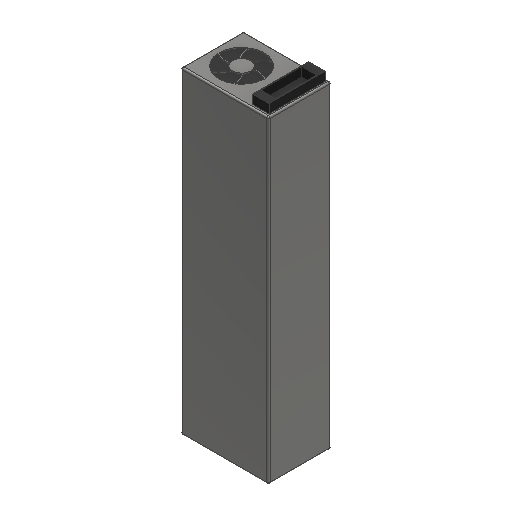
# Autodesk Inventor part: COTS_HP_DPS-600PB_PSU
Saved by Autodesk Inventor 2026.1 (Build 301233000, 233)
## iProperties
Created: 2016-06-20
Part Number: COTS_HP_DPS-600PB_PSU
Material: Ogólny
Document SubType Name: Modeling
Designer: Andrzej
Density: 1 g/cm^3
Appearance: Anodowana - jasnoszara
Author: Andrzej
Autodesk Inventor part; units mm, degrees
(part 1 of 2)
ref_plane "YZ Plane" through (0, 0, 0) normal (1, 0, 0) x (0, 1, 0)
ref_plane "XZ Plane" through (0, 0, 0) normal (0, 1, 0) x (-1, 0, 0)
ref_plane "XY Plane" through (0, 0, 0) normal (0, 0, 1) x (1, 0, 0)
sketch "Szkic1" plane through (0, 0, 0) normal (0, 0, 1) x (1, 0, 0)
  line L0 (-0.3998, -24.5096) -> (77.1002, -24.5096)
  line L1 (77.1002, -24.5096) -> (77.1002, -80.0096)
  line L2 (77.1002, -80.0096) -> (-0.3998, -80.0096)
  line L3 (-0.3998, -80.0096) -> (-0.3998, -24.5096)
  point P0 (0, 0)
  dimension "d0" = 77.5
  dimension "d1" = 55.5
  constraints: 8 end point, 2 parallel, 1 horizontal, 1 perpendicular
  measures "d0" distance of L1.end L2.end
  measures "d1" distance of L0.end L1.end
extrude "Wyciągnięcie proste1" add sketch "Szkic1" along normal blind 281.5
fillet "Zaokrąglenie1" radius 1.5 12 edges at (77.1002, -24.5096, 140.75) (77.1002, -80.0096, 140.75) (-0.3998, -24.5096, 140.75) (38.3502, -24.5096, 0) (38.3502, -80.0096, 0) (77.1002, -52.2596, 0) (-0.3998, -52.2596, 0) (38.3502, -24.5096, 281.5) (77.1002, -52.2596, 281.5) (38.3502, -80.0096, 281.5) (-0.3998, -52.2596, 281.5) (-0.3998, -80.0096, 140.75)
sketch "Szkic2" plane through (0, 0, 0) normal (0, 0, -1) x (-1, 0, 0)
  line L0 (-34.6002, -49.0096) -> (-3.6002, -49.0096)
  line L1 (-3.6002, -49.0096) -> (-3.6002, -73.0096)
  line L2 (-3.6002, -73.0096) -> (-34.6002, -73.0096)
  line L3 (-34.6002, -73.0096) -> (-34.6002, -49.0096)
  arc A0 (-75.6002, -24.5096) -> (-77.1002, -26.0096) centre (-75.6002, -26.0096) ccw projected
  line L4 (-77.1002, -78.5096) -> (-75.6002, -78.5096) projected
  line L5 (-75.6002, -78.5096) -> (-75.6002, -26.0096) projected
  line L6 (-75.6002, -26.0096) -> (-77.1002, -26.0096) projected
  line L7 (-77.1002, -26.0096) -> (-77.1002, -78.5096) projected
  line L8 (-75.6002, -24.5096) -> (-75.6002, -26.0096) projected
  line L9 (-75.6002, -26.0096) -> (-1.1002, -26.0096) projected
  line L10 (-1.1002, -26.0096) -> (-1.1002, -24.5096) projected
  line L11 (-1.1002, -24.5096) -> (-75.6002, -24.5096) projected
  line L12 (-1.1002, -80.0096) -> (-1.1002, -78.5096) projected
  line L13 (-1.1002, -78.5096) -> (-75.6002, -78.5096) projected
  line L14 (-75.6002, -78.5096) -> (-75.6002, -80.0096) projected
  line L15 (-75.6002, -80.0096) -> (-1.1002, -80.0096) projected
  arc A1 (-1.1002, -80.0096) -> (0.3998, -78.5096) centre (-1.1002, -78.5096) ccw projected
  line L16 (0.3998, -78.5096) -> (-1.1002, -78.5096) projected
  line L17 (0.3998, -78.5096) -> (0.3998, -26.0096) projected
  line L18 (-1.1002, -26.0096) -> (-1.1002, -78.5096) projected
  line L19 (0.3998, -26.0096) -> (-1.1002, -26.0096) projected
  line L20 (-1.1002, -26.0096) -> (-1.1002, -78.5096) projected
  line L21 (-1.1002, -78.5096) -> (0.3998, -78.5096) projected
  line L22 (0.3998, -78.5096) -> (0.3998, -26.0096) projected
  arc A2 (0.3998, -26.0096) -> (-1.1002, -24.5096) centre (-1.1002, -26.0096) ccw projected
  line L23 (-75.6002, -80.0096) -> (-75.6002, -78.5096) projected
  line L24 (-75.6002, -78.5096) -> (-75.6002, -80.0096) projected
  line L25 (-77.1002, -78.5096) -> (-75.6002, -78.5096) projected
  arc A3 (-77.1002, -78.5096) -> (-75.6002, -80.0096) centre (-75.6002, -78.5096) ccw projected
  circle A4 centre (-38.6002, -71.0096) radius 3.75
  circle A5 centre (-38.6002, -71.0096) radius 2.5
  line L26 (-31.6002, -53.0096) -> (-6.6002, -53.0096)
  line L27 (-31.6002, -69.0096) -> (-6.6002, -69.0096)
  line L28 (-31.6002, -53.0096) -> (-31.6002, -69.0096)
  line L29 (-6.6002, -53.0096) -> (-6.6002, -69.0096)
  line L30 (-70.6002, -30.3756) -> (-72.1002, -31.2416)
  line L31 (-72.1002, -31.2416) -> (-73.6002, -30.3756)
  line L32 (-73.6002, -30.3756) -> (-73.6002, -28.6435)
  line L33 (-73.6002, -28.6435) -> (-72.1002, -27.7775)
  line L34 (-72.1002, -27.7775) -> (-70.6002, -28.6435)
  line L35 (-70.6002, -28.6435) -> (-70.6002, -30.3756)
  line L36 (-68.1002, -31.2416) -> (-69.6002, -30.3756)
  line L37 (-66.6002, -30.3756) -> (-68.1002, -31.2416)
  line L38 (-69.6002, -30.3756) -> (-69.6002, -28.6435)
  line L39 (-66.6002, -28.6435) -> (-66.6002, -30.3756)
  line L40 (-69.6002, -28.6435) -> (-68.1002, -27.7775)
  line L41 (-68.1002, -27.7775) -> (-66.6002, -28.6435)
  line L42 (-64.1002, -31.2416) -> (-65.6002, -30.3756)
  line L43 (-62.6002, -30.3756) -> (-64.1002, -31.2416)
  line L44 (-65.6002, -30.3756) -> (-65.6002, -28.6435)
  line L45 (-62.6002, -28.6435) -> (-62.6002, -30.3756)
  line L46 (-65.6002, -28.6435) -> (-64.1002, -27.7775)
  line L47 (-64.1002, -27.7775) -> (-62.6002, -28.6435)
  line L48 (-60.1002, -31.2416) -> (-61.6002, -30.3756)
  line L49 (-58.6002, -30.3756) -> (-60.1002, -31.2416)
  line L50 (-61.6002, -30.3756) -> (-61.6002, -28.6435)
  line L51 (-58.6002, -28.6435) -> (-58.6002, -30.3756)
  line L52 (-61.6002, -28.6435) -> (-60.1002, -27.7775)
  line L53 (-60.1002, -27.7775) -> (-58.6002, -28.6435)
  line L54 (-56.1002, -31.2416) -> (-57.6002, -30.3756)
  line L55 (-54.6002, -30.3756) -> (-56.1002, -31.2416)
  line L56 (-57.6002, -30.3756) -> (-57.6002, -28.6435)
  line L57 (-54.6002, -28.6435) -> (-54.6002, -30.3756)
  line L58 (-57.6002, -28.6435) -> (-56.1002, -27.7775)
  line L59 (-56.1002, -27.7775) -> (-54.6002, -28.6435)
  line L60 (-52.1002, -31.2416) -> (-53.6002, -30.3756)
  line L61 (-50.6002, -30.3756) -> (-52.1002, -31.2416)
  line L62 (-53.6002, -30.3756) -> (-53.6002, -28.6435)
  line L63 (-50.6002, -28.6435) -> (-50.6002, -30.3756)
  line L64 (-53.6002, -28.6435) -> (-52.1002, -27.7775)
  line L65 (-52.1002, -27.7775) -> (-50.6002, -28.6435)
  line L66 (-48.1002, -31.2416) -> (-49.6002, -30.3756)
  line L67 (-46.6002, -30.3756) -> (-48.1002, -31.2416)
  line L68 (-49.6002, -30.3756) -> (-49.6002, -28.6435)
  line L69 (-46.6002, -28.6435) -> (-46.6002, -30.3756)
  line L70 (-49.6002, -28.6435) -> (-48.1002, -27.7775)
  line L71 (-48.1002, -27.7775) -> (-46.6002, -28.6435)
  line L72 (-44.1002, -31.2416) -> (-45.6002, -30.3756)
  line L73 (-42.6002, -30.3756) -> (-44.1002, -31.2416)
  line L74 (-45.6002, -30.3756) -> (-45.6002, -28.6435)
  line L75 (-42.6002, -28.6435) -> (-42.6002, -30.3756)
  line L76 (-45.6002, -28.6435) -> (-44.1002, -27.7775)
  line L77 (-44.1002, -27.7775) -> (-42.6002, -28.6435)
  line L78 (-40.1002, -31.2416) -> (-41.6002, -30.3756)
  line L79 (-38.6002, -30.3756) -> (-40.1002, -31.2416)
  line L80 (-41.6002, -30.3756) -> (-41.6002, -28.6435)
  line L81 (-38.6002, -28.6435) -> (-38.6002, -30.3756)
  line L82 (-41.6002, -28.6435) -> (-40.1002, -27.7775)
  line L83 (-40.1002, -27.7775) -> (-38.6002, -28.6435)
  line L84 (-36.1002, -31.2416) -> (-37.6002, -30.3756)
  line L85 (-34.6002, -30.3756) -> (-36.1002, -31.2416)
  line L86 (-37.6002, -30.3756) -> (-37.6002, -28.6435)
  line L87 (-34.6002, -28.6435) -> (-34.6002, -30.3756)
  line L88 (-37.6002, -28.6435) -> (-36.1002, -27.7775)
  line L89 (-36.1002, -27.7775) -> (-34.6002, -28.6435)
  line L90 (-32.1002, -31.2416) -> (-33.6002, -30.3756)
  line L91 (-30.6002, -30.3756) -> (-32.1002, -31.2416)
  line L92 (-33.6002, -30.3756) -> (-33.6002, -28.6435)
  line L93 (-30.6002, -28.6435) -> (-30.6002, -30.3756)
  line L94 (-33.6002, -28.6435) -> (-32.1002, -27.7775)
  line L95 (-32.1002, -27.7775) -> (-30.6002, -28.6435)
  line L96 (-28.1002, -31.2416) -> (-29.6002, -30.3756)
  line L97 (-26.6002, -30.3756) -> (-28.1002, -31.2416)
  line L98 (-29.6002, -30.3756) -> (-29.6002, -28.6435)
  line L99 (-26.6002, -28.6435) -> (-26.6002, -30.3756)
  line L100 (-29.6002, -28.6435) -> (-28.1002, -27.7775)
  line L101 (-28.1002, -27.7775) -> (-26.6002, -28.6435)
  line L102 (-24.1002, -31.2416) -> (-25.6002, -30.3756)
  line L103 (-22.6002, -30.3756) -> (-24.1002, -31.2416)
  line L104 (-25.6002, -30.3756) -> (-25.6002, -28.6435)
  line L105 (-22.6002, -28.6435) -> (-22.6002, -30.3756)
  line L106 (-25.6002, -28.6435) -> (-24.1002, -27.7775)
  line L107 (-24.1002, -27.7775) -> (-22.6002, -28.6435)
  line L108 (-20.1002, -31.2416) -> (-21.6002, -30.3756)
  line L109 (-18.6002, -30.3756) -> (-20.1002, -31.2416)
  line L110 (-21.6002, -30.3756) -> (-21.6002, -28.6435)
  line L111 (-18.6002, -28.6435) -> (-18.6002, -30.3756)
  line L112 (-21.6002, -28.6435) -> (-20.1002, -27.7775)
  line L113 (-20.1002, -27.7775) -> (-18.6002, -28.6435)
  line L114 (-16.1002, -31.2416) -> (-17.6002, -30.3756)
  line L115 (-14.6002, -30.3756) -> (-16.1002, -31.2416)
  line L116 (-17.6002, -30.3756) -> (-17.6002, -28.6435)
  line L117 (-14.6002, -28.6435) -> (-14.6002, -30.3756)
  line L118 (-17.6002, -28.6435) -> (-16.1002, -27.7775)
  line L119 (-16.1002, -27.7775) -> (-14.6002, -28.6435)
  line L120 (-12.1002, -31.2416) -> (-13.6002, -30.3756)
  line L121 (-10.6002, -30.3756) -> (-12.1002, -31.2416)
  line L122 (-13.6002, -30.3756) -> (-13.6002, -28.6435)
  line L123 (-10.6002, -28.6435) -> (-10.6002, -30.3756)
  line L124 (-13.6002, -28.6435) -> (-12.1002, -27.7775)
  line L125 (-12.1002, -27.7775) -> (-10.6002, -28.6435)
  line L126 (-8.1002, -31.2416) -> (-9.6002, -30.3756)
  line L127 (-6.6002, -30.3756) -> (-8.1002, -31.2416)
  line L128 (-9.6002, -30.3756) -> (-9.6002, -28.6435)
  line L129 (-6.6002, -28.6435) -> (-6.6002, -30.3756)
  line L130 (-9.6002, -28.6435) -> (-8.1002, -27.7775)
  line L131 (-8.1002, -27.7775) -> (-6.6002, -28.6435)
  line L132 (-72.1002, -35.2416) -> (-73.6002, -34.3756)
  line L133 (-70.6002, -34.3756) -> (-72.1002, -35.2416)
  line L134 (-73.6002, -34.3756) -> (-73.6002, -32.6435)
  line L135 (-70.6002, -32.6435) -> (-70.6002, -34.3756)
  line L136 (-73.6002, -32.6435) -> (-72.1002, -31.7775)
  line L137 (-72.1002, -31.7775) -> (-70.6002, -32.6435)
  line L138 (-68.1002, -35.2416) -> (-69.6002, -34.3756)
  line L139 (-66.6002, -34.3756) -> (-68.1002, -35.2416)
  line L140 (-69.6002, -34.3756) -> (-69.6002, -32.6435)
  line L141 (-66.6002, -32.6435) -> (-66.6002, -34.3756)
  line L142 (-69.6002, -32.6435) -> (-68.1002, -31.7775)
  line L143 (-68.1002, -31.7775) -> (-66.6002, -32.6435)
  line L144 (-64.1002, -35.2416) -> (-65.6002, -34.3756)
  line L145 (-62.6002, -34.3756) -> (-64.1002, -35.2416)
  line L146 (-65.6002, -34.3756) -> (-65.6002, -32.6435)
  line L147 (-62.6002, -32.6435) -> (-62.6002, -34.3756)
  line L148 (-65.6002, -32.6435) -> (-64.1002, -31.7775)
  line L149 (-64.1002, -31.7775) -> (-62.6002, -32.6435)
  line L150 (-60.1002, -35.2416) -> (-61.6002, -34.3756)
  line L151 (-58.6002, -34.3756) -> (-60.1002, -35.2416)
  line L152 (-61.6002, -34.3756) -> (-61.6002, -32.6435)
  line L153 (-58.6002, -32.6435) -> (-58.6002, -34.3756)
  line L154 (-61.6002, -32.6435) -> (-60.1002, -31.7775)
  line L155 (-60.1002, -31.7775) -> (-58.6002, -32.6435)
  line L156 (-56.1002, -35.2416) -> (-57.6002, -34.3756)
  line L157 (-54.6002, -34.3756) -> (-56.1002, -35.2416)
  line L158 (-57.6002, -34.3756) -> (-57.6002, -32.6435)
  line L159 (-54.6002, -32.6435) -> (-54.6002, -34.3756)
  line L160 (-57.6002, -32.6435) -> (-56.1002, -31.7775)
  line L161 (-56.1002, -31.7775) -> (-54.6002, -32.6435)
  line L162 (-52.1002, -35.2416) -> (-53.6002, -34.3756)
  line L163 (-50.6002, -34.3756) -> (-52.1002, -35.2416)
  line L164 (-53.6002, -34.3756) -> (-53.6002, -32.6435)
  line L165 (-50.6002, -32.6435) -> (-50.6002, -34.3756)
  line L166 (-53.6002, -32.6435) -> (-52.1002, -31.7775)
  line L167 (-52.1002, -31.7775) -> (-50.6002, -32.6435)
  line L168 (-48.1002, -35.2416) -> (-49.6002, -34.3756)
  line L169 (-46.6002, -34.3756) -> (-48.1002, -35.2416)
  line L170 (-49.6002, -34.3756) -> (-49.6002, -32.6435)
  line L171 (-46.6002, -32.6435) -> (-46.6002, -34.3756)
  line L172 (-49.6002, -32.6435) -> (-48.1002, -31.7775)
  line L173 (-48.1002, -31.7775) -> (-46.6002, -32.6435)
  line L174 (-44.1002, -35.2416) -> (-45.6002, -34.3756)
  line L175 (-42.6002, -34.3756) -> (-44.1002, -35.2416)
  line L176 (-45.6002, -34.3756) -> (-45.6002, -32.6435)
  line L177 (-42.6002, -32.6435) -> (-42.6002, -34.3756)
  line L178 (-45.6002, -32.6435) -> (-44.1002, -31.7775)
  line L179 (-44.1002, -31.7775) -> (-42.6002, -32.6435)
  line L180 (-40.1002, -35.2416) -> (-41.6002, -34.3756)
  line L181 (-38.6002, -34.3756) -> (-40.1002, -35.2416)
  line L182 (-41.6002, -34.3756) -> (-41.6002, -32.6435)
  line L183 (-38.6002, -32.6435) -> (-38.6002, -34.3756)
  line L184 (-41.6002, -32.6435) -> (-40.1002, -31.7775)
  line L185 (-40.1002, -31.7775) -> (-38.6002, -32.6435)
  line L186 (-36.1002, -35.2416) -> (-37.6002, -34.3756)
  line L187 (-34.6002, -34.3756) -> (-36.1002, -35.2416)
  line L188 (-37.6002, -34.3756) -> (-37.6002, -32.6435)
  line L189 (-34.6002, -32.6435) -> (-34.6002, -34.3756)
  line L190 (-37.6002, -32.6435) -> (-36.1002, -31.7775)
  line L191 (-36.1002, -31.7775) -> (-34.6002, -32.6435)
  line L192 (-32.1002, -35.2416) -> (-33.6002, -34.3756)
  line L193 (-30.6002, -34.3756) -> (-32.1002, -35.2416)
  line L194 (-33.6002, -34.3756) -> (-33.6002, -32.6435)
  line L195 (-30.6002, -32.6435) -> (-30.6002, -34.3756)
  line L196 (-33.6002, -32.6435) -> (-32.1002, -31.7775)
  line L197 (-32.1002, -31.7775) -> (-30.6002, -32.6435)
  line L198 (-28.1002, -35.2416) -> (-29.6002, -34.3756)
  line L199 (-26.6002, -34.3756) -> (-28.1002, -35.2416)
  line L200 (-29.6002, -34.3756) -> (-29.6002, -32.6435)
  line L201 (-26.6002, -32.6435) -> (-26.6002, -34.3756)
  line L202 (-29.6002, -32.6435) -> (-28.1002, -31.7775)
  line L203 (-28.1002, -31.7775) -> (-26.6002, -32.6435)
  line L204 (-24.1002, -35.2416) -> (-25.6002, -34.3756)
  line L205 (-22.6002, -34.3756) -> (-24.1002, -35.2416)
  line L206 (-25.6002, -34.3756) -> (-25.6002, -32.6435)
  line L207 (-22.6002, -32.6435) -> (-22.6002, -34.3756)
  line L208 (-25.6002, -32.6435) -> (-24.1002, -31.7775)
  line L209 (-24.1002, -31.7775) -> (-22.6002, -32.6435)
  line L210 (-20.1002, -35.2416) -> (-21.6002, -34.3756)
  line L211 (-18.6002, -34.3756) -> (-20.1002, -35.2416)
  line L212 (-21.6002, -34.3756) -> (-21.6002, -32.6435)
  line L213 (-18.6002, -32.6435) -> (-18.6002, -34.3756)
  line L214 (-21.6002, -32.6435) -> (-20.1002, -31.7775)
  line L215 (-20.1002, -31.7775) -> (-18.6002, -32.6435)
  line L216 (-16.1002, -35.2416) -> (-17.6002, -34.3756)
  line L217 (-14.6002, -34.3756) -> (-16.1002, -35.2416)
  line L218 (-17.6002, -34.3756) -> (-17.6002, -32.6435)
  line L219 (-14.6002, -32.6435) -> (-14.6002, -34.3756)
  line L220 (-17.6002, -32.6435) -> (-16.1002, -31.7775)
  line L221 (-16.1002, -31.7775) -> (-14.6002, -32.6435)
  line L222 (-12.1002, -35.2416) -> (-13.6002, -34.3756)
  line L223 (-10.6002, -34.3756) -> (-12.1002, -35.2416)
  line L224 (-13.6002, -34.3756) -> (-13.6002, -32.6435)
  line L225 (-10.6002, -32.6435) -> (-10.6002, -34.3756)
  line L226 (-13.6002, -32.6435) -> (-12.1002, -31.7775)
  line L227 (-12.1002, -31.7775) -> (-10.6002, -32.6435)
  line L228 (-8.1002, -35.2416) -> (-9.6002, -34.3756)
  line L229 (-6.6002, -34.3756) -> (-8.1002, -35.2416)
  line L230 (-9.6002, -34.3756) -> (-9.6002, -32.6435)
  line L231 (-6.6002, -32.6435) -> (-6.6002, -34.3756)
  line L232 (-9.6002, -32.6435) -> (-8.1002, -31.7775)
  line L233 (-8.1002, -31.7775) -> (-6.6002, -32.6435)
  line L234 (-72.1002, -39.2416) -> (-73.6002, -38.3756)
  line L235 (-70.6002, -38.3756) -> (-72.1002, -39.2416)
  line L236 (-73.6002, -38.3756) -> (-73.6002, -36.6435)
  line L237 (-70.6002, -36.6435) -> (-70.6002, -38.3756)
  line L238 (-73.6002, -36.6435) -> (-72.1002, -35.7775)
  line L239 (-72.1002, -35.7775) -> (-70.6002, -36.6435)
  line L240 (-68.1002, -39.2416) -> (-69.6002, -38.3756)
  line L241 (-66.6002, -38.3756) -> (-68.1002, -39.2416)
  line L242 (-69.6002, -38.3756) -> (-69.6002, -36.6435)
  line L243 (-66.6002, -36.6435) -> (-66.6002, -38.3756)
  line L244 (-69.6002, -36.6435) -> (-68.1002, -35.7775)
  line L245 (-68.1002, -35.7775) -> (-66.6002, -36.6435)
  line L246 (-64.1002, -39.2416) -> (-65.6002, -38.3756)
  line L247 (-62.6002, -38.3756) -> (-64.1002, -39.2416)
  line L248 (-65.6002, -38.3756) -> (-65.6002, -36.6435)
  line L249 (-62.6002, -36.6435) -> (-62.6002, -38.3756)
  line L250 (-65.6002, -36.6435) -> (-64.1002, -35.7775)
  line L251 (-64.1002, -35.7775) -> (-62.6002, -36.6435)
  line L252 (-60.1002, -39.2416) -> (-61.6002, -38.3756)
  line L253 (-58.6002, -38.3756) -> (-60.1002, -39.2416)
  line L254 (-61.6002, -38.3756) -> (-61.6002, -36.6435)
  line L255 (-58.6002, -36.6435) -> (-58.6002, -38.3756)
  line L256 (-61.6002, -36.6435) -> (-60.1002, -35.7775)
  line L257 (-60.1002, -35.7775) -> (-58.6002, -36.6435)
  line L258 (-56.1002, -39.2416) -> (-57.6002, -38.3756)
  line L259 (-54.6002, -38.3756) -> (-56.1002, -39.2416)
  line L260 (-57.6002, -38.3756) -> (-57.6002, -36.6435)
  line L261 (-54.6002, -36.6435) -> (-54.6002, -38.3756)
  line L262 (-57.6002, -36.6435) -> (-56.1002, -35.7775)
  line L263 (-56.1002, -35.7775) -> (-54.6002, -36.6435)
  line L264 (-52.1002, -39.2416) -> (-53.6002, -38.3756)
  line L265 (-50.6002, -38.3756) -> (-52.1002, -39.2416)
  line L266 (-53.6002, -38.3756) -> (-53.6002, -36.6435)
  line L267 (-50.6002, -36.6435) -> (-50.6002, -38.3756)
  line L268 (-53.6002, -36.6435) -> (-52.1002, -35.7775)
  line L269 (-52.1002, -35.7775) -> (-50.6002, -36.6435)
  line L270 (-48.1002, -39.2416) -> (-49.6002, -38.3756)
  line L271 (-46.6002, -38.3756) -> (-48.1002, -39.2416)
  line L272 (-49.6002, -38.3756) -> (-49.6002, -36.6435)
  line L273 (-46.6002, -36.6435) -> (-46.6002, -38.3756)
  line L274 (-49.6002, -36.6435) -> (-48.1002, -35.7775)
  line L275 (-48.1002, -35.7775) -> (-46.6002, -36.6435)
  line L276 (-44.1002, -39.2416) -> (-45.6002, -38.3756)
  line L277 (-42.6002, -38.3756) -> (-44.1002, -39.2416)
  line L278 (-45.6002, -38.3756) -> (-45.6002, -36.6435)
  line L279 (-42.6002, -36.6435) -> (-42.6002, -38.3756)
  line L280 (-45.6002, -36.6435) -> (-44.1002, -35.7775)
  line L281 (-44.1002, -35.7775) -> (-42.6002, -36.6435)
  line L282 (-40.1002, -39.2416) -> (-41.6002, -38.3756)
  line L283 (-38.6002, -38.3756) -> (-40.1002, -39.2416)
  line L284 (-41.6002, -38.3756) -> (-41.6002, -36.6435)
  line L285 (-38.6002, -36.6435) -> (-38.6002, -38.3756)
  line L286 (-41.6002, -36.6435) -> (-40.1002, -35.7775)
  line L287 (-40.1002, -35.7775) -> (-38.6002, -36.6435)
  line L288 (-36.1002, -39.2416) -> (-37.6002, -38.3756)
  line L289 (-34.6002, -38.3756) -> (-36.1002, -39.2416)
  line L290 (-37.6002, -38.3756) -> (-37.6002, -36.6435)
  line L291 (-34.6002, -36.6435) -> (-34.6002, -38.3756)
  line L292 (-37.6002, -36.6435) -> (-36.1002, -35.7775)
  line L293 (-36.1002, -35.7775) -> (-34.6002, -36.6435)
  line L294 (-32.1002, -39.2416) -> (-33.6002, -38.3756)
  line L295 (-30.6002, -38.3756) -> (-32.1002, -39.2416)
  line L296 (-33.6002, -38.3756) -> (-33.6002, -36.6435)
  line L297 (-30.6002, -36.6435) -> (-30.6002, -38.3756)
  line L298 (-33.6002, -36.6435) -> (-32.1002, -35.7775)
  line L299 (-32.1002, -35.7775) -> (-30.6002, -36.6435)
  line L300 (-28.1002, -39.2416) -> (-29.6002, -38.3756)
  line L301 (-26.6002, -38.3756) -> (-28.1002, -39.2416)
  line L302 (-29.6002, -38.3756) -> (-29.6002, -36.6435)
  line L303 (-26.6002, -36.6435) -> (-26.6002, -38.3756)
  line L304 (-29.6002, -36.6435) -> (-28.1002, -35.7775)
  line L305 (-28.1002, -35.7775) -> (-26.6002, -36.6435)
  line L306 (-24.1002, -39.2416) -> (-25.6002, -38.3756)
  line L307 (-22.6002, -38.3756) -> (-24.1002, -39.2416)
  line L308 (-25.6002, -38.3756) -> (-25.6002, -36.6435)
  line L309 (-22.6002, -36.6435) -> (-22.6002, -38.3756)
  line L310 (-25.6002, -36.6435) -> (-24.1002, -35.7775)
  line L311 (-24.1002, -35.7775) -> (-22.6002, -36.6435)
  line L312 (-20.1002, -39.2416) -> (-21.6002, -38.3756)
  line L313 (-18.6002, -38.3756) -> (-20.1002, -39.2416)
  line L314 (-21.6002, -38.3756) -> (-21.6002, -36.6435)
  line L315 (-18.6002, -36.6435) -> (-18.6002, -38.3756)
  line L316 (-21.6002, -36.6435) -> (-20.1002, -35.7775)
  line L317 (-20.1002, -35.7775) -> (-18.6002, -36.6435)
  line L318 (-16.1002, -39.2416) -> (-17.6002, -38.3756)
  line L319 (-14.6002, -38.3756) -> (-16.1002, -39.2416)
  line L320 (-17.6002, -38.3756) -> (-17.6002, -36.6435)
  line L321 (-14.6002, -36.6435) -> (-14.6002, -38.3756)
  line L322 (-17.6002, -36.6435) -> (-16.1002, -35.7775)
  line L323 (-16.1002, -35.7775) -> (-14.6002, -36.6435)
  line L324 (-12.1002, -39.2416) -> (-13.6002, -38.3756)
  line L325 (-10.6002, -38.3756) -> (-12.1002, -39.2416)
  line L326 (-13.6002, -38.3756) -> (-13.6002, -36.6435)
  line L327 (-10.6002, -36.6435) -> (-10.6002, -38.3756)
  line L328 (-13.6002, -36.6435) -> (-12.1002, -35.7775)
  line L329 (-12.1002, -35.7775) -> (-10.6002, -36.6435)
  line L330 (-8.1002, -39.2416) -> (-9.6002, -38.3756)
  line L331 (-6.6002, -38.3756) -> (-8.1002, -39.2416)
  line L332 (-9.6002, -38.3756) -> (-9.6002, -36.6435)
  line L333 (-6.6002, -36.6435) -> (-6.6002, -38.3756)
  line L334 (-9.6002, -36.6435) -> (-8.1002, -35.7775)
  line L335 (-8.1002, -35.7775) -> (-6.6002, -36.6435)
  line L336 (-72.1002, -43.2416) -> (-73.6002, -42.3756)
  line L337 (-70.6002, -42.3756) -> (-72.1002, -43.2416)
  line L338 (-73.6002, -42.3756) -> (-73.6002, -40.6435)
  line L339 (-70.6002, -40.6435) -> (-70.6002, -42.3756)
  line L340 (-73.6002, -40.6435) -> (-72.1002, -39.7775)
  line L341 (-72.1002, -39.7775) -> (-70.6002, -40.6435)
  line L342 (-68.1002, -43.2416) -> (-69.6002, -42.3756)
  line L343 (-66.6002, -42.3756) -> (-68.1002, -43.2416)
  line L344 (-69.6002, -42.3756) -> (-69.6002, -40.6435)
  line L345 (-66.6002, -40.6435) -> (-66.6002, -42.3756)
  line L346 (-69.6002, -40.6435) -> (-68.1002, -39.7775)
  line L347 (-68.1002, -39.7775) -> (-66.6002, -40.6435)
  line L348 (-64.1002, -43.2416) -> (-65.6002, -42.3756)
  line L349 (-62.6002, -42.3756) -> (-64.1002, -43.2416)
  line L350 (-65.6002, -42.3756) -> (-65.6002, -40.6435)
  line L351 (-62.6002, -40.6435) -> (-62.6002, -42.3756)
  line L352 (-65.6002, -40.6435) -> (-64.1002, -39.7775)
  line L353 (-64.1002, -39.7775) -> (-62.6002, -40.6435)
  line L354 (-60.1002, -43.2416) -> (-61.6002, -42.3756)
  line L355 (-58.6002, -42.3756) -> (-60.1002, -43.2416)
  line L356 (-61.6002, -42.3756) -> (-61.6002, -40.6435)
  line L357 (-58.6002, -40.6435) -> (-58.6002, -42.3756)
  line L358 (-61.6002, -40.6435) -> (-60.1002, -39.7775)
  line L359 (-60.1002, -39.7775) -> (-58.6002, -40.6435)
  line L360 (-56.1002, -43.2416) -> (-57.6002, -42.3756)
  line L361 (-54.6002, -42.3756) -> (-56.1002, -43.2416)
  line L362 (-57.6002, -42.3756) -> (-57.6002, -40.6435)
  line L363 (-54.6002, -40.6435) -> (-54.6002, -42.3756)
  line L364 (-57.6002, -40.6435) -> (-56.1002, -39.7775)
  line L365 (-56.1002, -39.7775) -> (-54.6002, -40.6435)
  line L366 (-52.1002, -43.2416) -> (-53.6002, -42.3756)
  line L367 (-50.6002, -42.3756) -> (-52.1002, -43.2416)
  line L368 (-53.6002, -42.3756) -> (-53.6002, -40.6435)
  line L369 (-50.6002, -40.6435) -> (-50.6002, -42.3756)
  line L370 (-53.6002, -40.6435) -> (-52.1002, -39.7775)
  line L371 (-52.1002, -39.7775) -> (-50.6002, -40.6435)
  line L372 (-48.1002, -43.2416) -> (-49.6002, -42.3756)
  line L373 (-46.6002, -42.3756) -> (-48.1002, -43.2416)
  line L374 (-49.6002, -42.3756) -> (-49.6002, -40.6435)
  line L375 (-46.6002, -40.6435) -> (-46.6002, -42.3756)
  line L376 (-49.6002, -40.6435) -> (-48.1002, -39.7775)
  line L377 (-48.1002, -39.7775) -> (-46.6002, -40.6435)
  line L378 (-44.1002, -43.2416) -> (-45.6002, -42.3756)
  line L379 (-42.6002, -42.3756) -> (-44.1002, -43.2416)
  line L380 (-45.6002, -42.3756) -> (-45.6002, -40.6435)
  line L381 (-42.6002, -40.6435) -> (-42.6002, -42.3756)
  line L382 (-45.6002, -40.6435) -> (-44.1002, -39.7775)
  line L383 (-44.1002, -39.7775) -> (-42.6002, -40.6435)
  line L384 (-40.1002, -43.2416) -> (-41.6002, -42.3756)
  line L385 (-38.6002, -42.3756) -> (-40.1002, -43.2416)
  line L386 (-41.6002, -42.3756) -> (-41.6002, -40.6435)
  line L387 (-38.6002, -40.6435) -> (-38.6002, -42.3756)
  line L388 (-41.6002, -40.6435) -> (-40.1002, -39.7775)
  line L389 (-40.1002, -39.7775) -> (-38.6002, -40.6435)
  line L390 (-36.1002, -43.2416) -> (-37.6002, -42.3756)
  line L391 (-34.6002, -42.3756) -> (-36.1002, -43.2416)
  line L392 (-37.6002, -42.3756) -> (-37.6002, -40.6435)
  line L393 (-34.6002, -40.6435) -> (-34.6002, -42.3756)
  line L394 (-37.6002, -40.6435) -> (-36.1002, -39.7775)
  line L395 (-36.1002, -39.7775) -> (-34.6002, -40.6435)
  line L396 (-32.1002, -43.2416) -> (-33.6002, -42.3756)
  line L397 (-30.6002, -42.3756) -> (-32.1002, -43.2416)
  line L398 (-33.6002, -42.3756) -> (-33.6002, -40.6435)
  line L399 (-30.6002, -40.6435) -> (-30.6002, -42.3756)
  line L400 (-33.6002, -40.6435) -> (-32.1002, -39.7775)
  line L401 (-32.1002, -39.7775) -> (-30.6002, -40.6435)
  line L402 (-28.1002, -43.2416) -> (-29.6002, -42.3756)
  line L403 (-26.6002, -42.3756) -> (-28.1002, -43.2416)
  line L404 (-29.6002, -42.3756) -> (-29.6002, -40.6435)
  line L405 (-26.6002, -40.6435) -> (-26.6002, -42.3756)
  line L406 (-29.6002, -40.6435) -> (-28.1002, -39.7775)
  line L407 (-28.1002, -39.7775) -> (-26.6002, -40.6435)
  line L408 (-24.1002, -43.2416) -> (-25.6002, -42.3756)
  line L409 (-22.6002, -42.3756) -> (-24.1002, -43.2416)
  line L410 (-25.6002, -42.3756) -> (-25.6002, -40.6435)
  line L411 (-22.6002, -40.6435) -> (-22.6002, -42.3756)
  line L412 (-25.6002, -40.6435) -> (-24.1002, -39.7775)
  line L413 (-24.1002, -39.7775) -> (-22.6002, -40.6435)
  line L414 (-20.1002, -43.2416) -> (-21.6002, -42.3756)
  line L415 (-18.6002, -42.3756) -> (-20.1002, -43.2416)
  line L416 (-21.6002, -42.3756) -> (-21.6002, -40.6435)
  line L417 (-18.6002, -40.6435) -> (-18.6002, -42.3756)
  line L418 (-21.6002, -40.6435) -> (-20.1002, -39.7775)
  line L419 (-20.1002, -39.7775) -> (-18.6002, -40.6435)
  line L420 (-16.1002, -43.2416) -> (-17.6002, -42.3756)
  line L421 (-14.6002, -42.3756) -> (-16.1002, -43.2416)
  line L422 (-17.6002, -42.3756) -> (-17.6002, -40.6435)
  line L423 (-14.6002, -40.6435) -> (-14.6002, -42.3756)
  line L424 (-17.6002, -40.6435) -> (-16.1002, -39.7775)
  line L425 (-16.1002, -39.7775) -> (-14.6002, -40.6435)
  line L426 (-12.1002, -43.2416) -> (-13.6002, -42.3756)
  line L427 (-10.6002, -42.3756) -> (-12.1002, -43.2416)
  line L428 (-13.6002, -42.3756) -> (-13.6002, -40.6435)
  line L429 (-10.6002, -40.6435) -> (-10.6002, -42.3756)
  line L430 (-13.6002, -40.6435) -> (-12.1002, -39.7775)
  line L431 (-12.1002, -39.7775) -> (-10.6002, -40.6435)
  line L432 (-8.1002, -43.2416) -> (-9.6002, -42.3756)
  line L433 (-6.6002, -42.3756) -> (-8.1002, -43.2416)
  line L434 (-9.6002, -42.3756) -> (-9.6002, -40.6435)
  line L435 (-6.6002, -40.6435) -> (-6.6002, -42.3756)
  line L436 (-9.6002, -40.6435) -> (-8.1002, -39.7775)
  line L437 (-8.1002, -39.7775) -> (-6.6002, -40.6435)
  line L438 (-72.1002, -47.2416) -> (-73.6002, -46.3756)
  line L439 (-70.6002, -46.3756) -> (-72.1002, -47.2416)
  line L440 (-73.6002, -46.3756) -> (-73.6002, -44.6435)
  line L441 (-70.6002, -44.6435) -> (-70.6002, -46.3756)
  line L442 (-73.6002, -44.6435) -> (-72.1002, -43.7775)
  line L443 (-72.1002, -43.7775) -> (-70.6002, -44.6435)
  line L444 (-68.1002, -47.2416) -> (-69.6002, -46.3756)
  line L445 (-66.6002, -46.3756) -> (-68.1002, -47.2416)
  line L446 (-69.6002, -46.3756) -> (-69.6002, -44.6435)
  line L447 (-66.6002, -44.6435) -> (-66.6002, -46.3756)
  line L448 (-69.6002, -44.6435) -> (-68.1002, -43.7775)
  line L449 (-68.1002, -43.7775) -> (-66.6002, -44.6435)
  line L450 (-64.1002, -47.2416) -> (-65.6002, -46.3756)
  line L451 (-62.6002, -46.3756) -> (-64.1002, -47.2416)
  line L452 (-65.6002, -46.3756) -> (-65.6002, -44.6435)
  line L453 (-62.6002, -44.6435) -> (-62.6002, -46.3756)
  line L454 (-65.6002, -44.6435) -> (-64.1002, -43.7775)
  line L455 (-64.1002, -43.7775) -> (-62.6002, -44.6435)
  line L456 (-60.1002, -47.2416) -> (-61.6002, -46.3756)
  line L457 (-58.6002, -46.3756) -> (-60.1002, -47.2416)
  line L458 (-61.6002, -46.3756) -> (-61.6002, -44.6435)
  line L459 (-58.6002, -44.6435) -> (-58.6002, -46.3756)
  line L460 (-61.6002, -44.6435) -> (-60.1002, -43.7775)
  line L461 (-60.1002, -43.7775) -> (-58.6002, -44.6435)
  line L462 (-56.1002, -47.2416) -> (-57.6002, -46.3756)
  line L463 (-54.6002, -46.3756) -> (-56.1002, -47.2416)
  line L464 (-57.6002, -46.3756) -> (-57.6002, -44.6435)
  line L465 (-54.6002, -44.6435) -> (-54.6002, -46.3756)
  line L466 (-57.6002, -44.6435) -> (-56.1002, -43.7775)
  line L467 (-56.1002, -43.7775) -> (-54.6002, -44.6435)
  line L468 (-52.1002, -47.2416) -> (-53.6002, -46.3756)
  line L469 (-50.6002, -46.3756) -> (-52.1002, -47.2416)
  line L470 (-53.6002, -46.3756) -> (-53.6002, -44.6435)
  line L471 (-50.6002, -44.6435) -> (-50.6002, -46.3756)
  line L472 (-53.6002, -44.6435) -> (-52.1002, -43.7775)
  line L473 (-52.1002, -43.7775) -> (-50.6002, -44.6435)
  line L474 (-48.1002, -47.2416) -> (-49.6002, -46.3756)
  line L475 (-46.6002, -46.3756) -> (-48.1002, -47.2416)
  line L476 (-49.6002, -46.3756) -> (-49.6002, -44.6435)
  line L477 (-46.6002, -44.6435) -> (-46.6002, -46.3756)
  line L478 (-49.6002, -44.6435) -> (-48.1002, -43.7775)
  line L479 (-48.1002, -43.7775) -> (-46.6002, -44.6435)
  line L480 (-44.1002, -47.2416) -> (-45.6002, -46.3756)
  line L481 (-42.6002, -46.3756) -> (-44.1002, -47.2416)
  line L482 (-45.6002, -46.3756) -> (-45.6002, -44.6435)
  line L483 (-42.6002, -44.6435) -> (-42.6002, -46.3756)
  line L484 (-45.6002, -44.6435) -> (-44.1002, -43.7775)
  line L485 (-44.1002, -43.7775) -> (-42.6002, -44.6435)
  line L486 (-40.1002, -47.2416) -> (-41.6002, -46.3756)
  line L487 (-38.6002, -46.3756) -> (-40.1002, -47.2416)
  line L488 (-41.6002, -46.3756) -> (-41.6002, -44.6435)
  line L489 (-38.6002, -44.6435) -> (-38.6002, -46.3756)
  line L490 (-41.6002, -44.6435) -> (-40.1002, -43.7775)
  line L491 (-40.1002, -43.7775) -> (-38.6002, -44.6435)
  line L492 (-36.1002, -47.2416) -> (-37.6002, -46.3756)
  line L493 (-34.6002, -46.3756) -> (-36.1002, -47.2416)
  line L494 (-37.6002, -46.3756) -> (-37.6002, -44.6435)
  line L495 (-34.6002, -44.6435) -> (-34.6002, -46.3756)
  line L496 (-37.6002, -44.6435) -> (-36.1002, -43.7775)
  line L497 (-36.1002, -43.7775) -> (-34.6002, -44.6435)
  line L498 (-32.1002, -47.2416) -> (-33.6002, -46.3756)
  line L499 (-30.6002, -46.3756) -> (-32.1002, -47.2416)
  line L500 (-33.6002, -46.3756) -> (-33.6002, -44.6435)
  line L501 (-30.6002, -44.6435) -> (-30.6002, -46.3756)
  line L502 (-33.6002, -44.6435) -> (-32.1002, -43.7775)
  line L503 (-32.1002, -43.7775) -> (-30.6002, -44.6435)
  line L504 (-28.1002, -47.2416) -> (-29.6002, -46.3756)
  line L505 (-26.6002, -46.3756) -> (-28.1002, -47.2416)
  line L506 (-29.6002, -46.3756) -> (-29.6002, -44.6435)
  line L507 (-26.6002, -44.6435) -> (-26.6002, -46.3756)
  line L508 (-29.6002, -44.6435) -> (-28.1002, -43.7775)
  line L509 (-28.1002, -43.7775) -> (-26.6002, -44.6435)
  line L510 (-24.1002, -47.2416) -> (-25.6002, -46.3756)
  line L511 (-22.6002, -46.3756) -> (-24.1002, -47.2416)
  line L512 (-25.6002, -46.3756) -> (-25.6002, -44.6435)
  line L513 (-22.6002, -44.6435) -> (-22.6002, -46.3756)
  line L514 (-25.6002, -44.6435) -> (-24.1002, -43.7775)
  line L515 (-24.1002, -43.7775) -> (-22.6002, -44.6435)
  line L516 (-20.1002, -47.2416) -> (-21.6002, -46.3756)
  line L517 (-18.6002, -46.3756) -> (-20.1002, -47.2416)
  line L518 (-21.6002, -46.3756) -> (-21.6002, -44.6435)
  line L519 (-18.6002, -44.6435) -> (-18.6002, -46.3756)
  line L520 (-21.6002, -44.6435) -> (-20.1002, -43.7775)
  line L521 (-20.1002, -43.7775) -> (-18.6002, -44.6435)
  line L522 (-16.1002, -47.2416) -> (-17.6002, -46.3756)
  line L523 (-14.6002, -46.3756) -> (-16.1002, -47.2416)
  line L524 (-17.6002, -46.3756) -> (-17.6002, -44.6435)
  line L525 (-14.6002, -44.6435) -> (-14.6002, -46.3756)
  line L526 (-17.6002, -44.6435) -> (-16.1002, -43.7775)
  line L527 (-16.1002, -43.7775) -> (-14.6002, -44.6435)
  line L528 (-12.1002, -47.2416) -> (-13.6002, -46.3756)
  line L529 (-10.6002, -46.3756) -> (-12.1002, -47.2416)
  line L530 (-13.6002, -46.3756) -> (-13.6002, -44.6435)
  line L531 (-10.6002, -44.6435) -> (-10.6002, -46.3756)
  line L532 (-13.6002, -44.6435) -> (-12.1002, -43.7775)
  line L533 (-12.1002, -43.7775) -> (-10.6002, -44.6435)
  line L534 (-8.1002, -47.2416) -> (-9.6002, -46.3756)
  line L535 (-6.6002, -46.3756) -> (-8.1002, -47.2416)
  line L536 (-9.6002, -46.3756) -> (-9.6002, -44.6435)
  line L537 (-6.6002, -44.6435) -> (-6.6002, -46.3756)
  line L538 (-9.6002, -44.6435) -> (-8.1002, -43.7775)
  line L539 (-8.1002, -43.7775) -> (-6.6002, -44.6435)
  line L540 (-66.6002, -44.6435) -> (-66.6002, -46.3756)
  line L541 (-68.1002, -43.7775) -> (-66.6002, -44.6435)
  line L542 (-66.6002, -46.3756) -> (-68.1002, -47.2416)
  line L543 (-69.6002, -44.6435) -> (-68.1002, -43.7775)
  line L544 (-68.1002, -47.2416) -> (-69.6002, -46.3756)
  line L545 (-69.6002, -46.3756) -> (-69.6002, -44.6435)
  line L546 (-62.6002, -44.6435) -> (-62.6002, -46.3756)
  line L547 (-64.1002, -43.7775) -> (-62.6002, -44.6435)
  line L548 (-62.6002, -46.3756) -> (-64.1002, -47.2416)
  line L549 (-65.6002, -44.6435) -> (-64.1002, -43.7775)
  line L550 (-64.1002, -47.2416) -> (-65.6002, -46.3756)
  line L551 (-65.6002, -46.3756) -> (-65.6002, -44.6435)
  line L552 (-58.6002, -44.6435) -> (-58.6002, -46.3756)
  line L553 (-60.1002, -43.7775) -> (-58.6002, -44.6435)
  line L554 (-58.6002, -46.3756) -> (-60.1002, -47.2416)
  line L555 (-61.6002, -44.6435) -> (-60.1002, -43.7775)
  line L556 (-60.1002, -47.2416) -> (-61.6002, -46.3756)
  line L557 (-61.6002, -46.3756) -> (-61.6002, -44.6435)
  line L558 (-54.6002, -44.6435) -> (-54.6002, -46.3756)
  line L559 (-56.1002, -43.7775) -> (-54.6002, -44.6435)
  line L560 (-54.6002, -46.3756) -> (-56.1002, -47.2416)
  line L561 (-57.6002, -44.6435) -> (-56.1002, -43.7775)
  line L562 (-56.1002, -47.2416) -> (-57.6002, -46.3756)
  line L563 (-57.6002, -46.3756) -> (-57.6002, -44.6435)
  line L564 (-50.6002, -44.6435) -> (-50.6002, -46.3756)
  line L565 (-52.1002, -43.7775) -> (-50.6002, -44.6435)
  line L566 (-50.6002, -46.3756) -> (-52.1002, -47.2416)
  line L567 (-53.6002, -44.6435) -> (-52.1002, -43.7775)
  line L568 (-52.1002, -47.2416) -> (-53.6002, -46.3756)
  line L569 (-53.6002, -46.3756) -> (-53.6002, -44.6435)
  line L570 (-46.6002, -44.6435) -> (-46.6002, -46.3756)
  line L571 (-48.1002, -43.7775) -> (-46.6002, -44.6435)
  line L572 (-46.6002, -46.3756) -> (-48.1002, -47.2416)
  line L573 (-49.6002, -44.6435) -> (-48.1002, -43.7775)
  line L574 (-48.1002, -47.2416) -> (-49.6002, -46.3756)
  line L575 (-49.6002, -46.3756) -> (-49.6002, -44.6435)
  line L576 (-42.6002, -44.6435) -> (-42.6002, -46.3756)
  line L577 (-44.1002, -43.7775) -> (-42.6002, -44.6435)
  line L578 (-42.6002, -46.3756) -> (-44.1002, -47.2416)
  line L579 (-45.6002, -44.6435) -> (-44.1002, -43.7775)
  line L580 (-44.1002, -47.2416) -> (-45.6002, -46.3756)
  line L581 (-45.6002, -46.3756) -> (-45.6002, -44.6435)
  line L582 (-38.6002, -44.6435) -> (-38.6002, -46.3756)
  line L583 (-40.1002, -43.7775) -> (-38.6002, -44.6435)
  line L584 (-38.6002, -46.3756) -> (-40.1002, -47.2416)
  line L585 (-41.6002, -44.6435) -> (-40.1002, -43.7775)
  line L586 (-40.1002, -47.2416) -> (-41.6002, -46.3756)
  line L587 (-41.6002, -46.3756) -> (-41.6002, -44.6435)
  line L588 (-70.6002, -48.6435) -> (-70.6002, -50.3756)
  line L589 (-72.1002, -47.7775) -> (-70.6002, -48.6435)
  line L590 (-70.6002, -50.3756) -> (-72.1002, -51.2416)
  line L591 (-73.6002, -48.6435) -> (-72.1002, -47.7775)
  line L592 (-72.1002, -51.2416) -> (-73.6002, -50.3756)
  line L593 (-73.6002, -50.3756) -> (-73.6002, -48.6435)
  line L594 (-66.6002, -48.6435) -> (-66.6002, -50.3756)
  line L595 (-68.1002, -47.7775) -> (-66.6002, -48.6435)
  line L596 (-66.6002, -50.3756) -> (-68.1002, -51.2416)
  line L597 (-69.6002, -48.6435) -> (-68.1002, -47.7775)
  line L598 (-68.1002, -51.2416) -> (-69.6002, -50.3756)
  line L599 (-69.6002, -50.3756) -> (-69.6002, -48.6435)
  line L600 (-62.6002, -48.6435) -> (-62.6002, -50.3756)
  line L601 (-64.1002, -47.7775) -> (-62.6002, -48.6435)
  line L602 (-62.6002, -50.3756) -> (-64.1002, -51.2416)
  line L603 (-65.6002, -48.6435) -> (-64.1002, -47.7775)
  line L604 (-64.1002, -51.2416) -> (-65.6002, -50.3756)
  line L605 (-65.6002, -50.3756) -> (-65.6002, -48.6435)
  line L606 (-58.6002, -48.6435) -> (-58.6002, -50.3756)
  line L607 (-60.1002, -47.7775) -> (-58.6002, -48.6435)
  line L608 (-58.6002, -50.3756) -> (-60.1002, -51.2416)
  line L609 (-61.6002, -48.6435) -> (-60.1002, -47.7775)
  line L610 (-60.1002, -51.2416) -> (-61.6002, -50.3756)
  line L611 (-61.6002, -50.3756) -> (-61.6002, -48.6435)
  line L612 (-54.6002, -48.6435) -> (-54.6002, -50.3756)
  line L613 (-56.1002, -47.7775) -> (-54.6002, -48.6435)
  line L614 (-54.6002, -50.3756) -> (-56.1002, -51.2416)
  line L615 (-57.6002, -48.6435) -> (-56.1002, -47.7775)
  line L616 (-56.1002, -51.2416) -> (-57.6002, -50.3756)
  line L617 (-57.6002, -50.3756) -> (-57.6002, -48.6435)
  line L618 (-50.6002, -48.6435) -> (-50.6002, -50.3756)
  line L619 (-52.1002, -47.7775) -> (-50.6002, -48.6435)
  line L620 (-50.6002, -50.3756) -> (-52.1002, -51.2416)
  line L621 (-53.6002, -48.6435) -> (-52.1002, -47.7775)
  line L622 (-52.1002, -51.2416) -> (-53.6002, -50.3756)
  line L623 (-53.6002, -50.3756) -> (-53.6002, -48.6435)
  line L624 (-46.6002, -48.6435) -> (-46.6002, -50.3756)
  line L625 (-48.1002, -47.7775) -> (-46.6002, -48.6435)
  line L626 (-46.6002, -50.3756) -> (-48.1002, -51.2416)
  line L627 (-49.6002, -48.6435) -> (-48.1002, -47.7775)
  line L628 (-48.1002, -51.2416) -> (-49.6002, -50.3756)
  line L629 (-49.6002, -50.3756) -> (-49.6002, -48.6435)
  line L630 (-42.6002, -48.6435) -> (-42.6002, -50.3756)
  line L631 (-44.1002, -47.7775) -> (-42.6002, -48.6435)
  line L632 (-42.6002, -50.3756) -> (-44.1002, -51.2416)
  line L633 (-45.6002, -48.6435) -> (-44.1002, -47.7775)
  line L634 (-44.1002, -51.2416) -> (-45.6002, -50.3756)
  line L635 (-45.6002, -50.3756) -> (-45.6002, -48.6435)
  line L636 (-38.6002, -48.6435) -> (-38.6002, -50.3756)
  line L637 (-40.1002, -47.7775) -> (-38.6002, -48.6435)
  line L638 (-38.6002, -50.3756) -> (-40.1002, -51.2416)
  line L639 (-41.6002, -48.6435) -> (-40.1002, -47.7775)
  line L640 (-40.1002, -51.2416) -> (-41.6002, -50.3756)
  line L641 (-41.6002, -50.3756) -> (-41.6002, -48.6435)
  line L642 (-70.6002, -52.6435) -> (-70.6002, -54.3756)
  line L643 (-72.1002, -51.7775) -> (-70.6002, -52.6435)
  line L644 (-70.6002, -54.3756) -> (-72.1002, -55.2416)
  line L645 (-73.6002, -52.6435) -> (-72.1002, -51.7775)
  line L646 (-72.1002, -55.2416) -> (-73.6002, -54.3756)
  line L647 (-73.6002, -54.3756) -> (-73.6002, -52.6435)
  line L648 (-66.6002, -52.6435) -> (-66.6002, -54.3756)
  line L649 (-68.1002, -51.7775) -> (-66.6002, -52.6435)
  line L650 (-66.6002, -54.3756) -> (-68.1002, -55.2416)
  line L651 (-69.6002, -52.6435) -> (-68.1002, -51.7775)
  line L652 (-68.1002, -55.2416) -> (-69.6002, -54.3756)
  line L653 (-69.6002, -54.3756) -> (-69.6002, -52.6435)
  line L654 (-62.6002, -52.6435) -> (-62.6002, -54.3756)
  line L655 (-64.1002, -51.7775) -> (-62.6002, -52.6435)
  line L656 (-62.6002, -54.3756) -> (-64.1002, -55.2416)
  line L657 (-65.6002, -52.6435) -> (-64.1002, -51.7775)
  line L658 (-64.1002, -55.2416) -> (-65.6002, -54.3756)
  line L659 (-65.6002, -54.3756) -> (-65.6002, -52.6435)
  line L660 (-58.6002, -52.6435) -> (-58.6002, -54.3756)
  line L661 (-60.1002, -51.7775) -> (-58.6002, -52.6435)
  line L662 (-58.6002, -54.3756) -> (-60.1002, -55.2416)
  line L663 (-61.6002, -52.6435) -> (-60.1002, -51.7775)
  line L664 (-60.1002, -55.2416) -> (-61.6002, -54.3756)
  line L665 (-61.6002, -54.3756) -> (-61.6002, -52.6435)
  line L666 (-54.6002, -52.6435) -> (-54.6002, -54.3756)
  line L667 (-56.1002, -51.7775) -> (-54.6002, -52.6435)
  line L668 (-54.6002, -54.3756) -> (-56.1002, -55.2416)
  line L669 (-57.6002, -52.6435) -> (-56.1002, -51.7775)
  line L670 (-56.1002, -55.2416) -> (-57.6002, -54.3756)
  line L671 (-57.6002, -54.3756) -> (-57.6002, -52.6435)
  line L672 (-50.6002, -52.6435) -> (-50.6002, -54.3756)
  line L673 (-52.1002, -51.7775) -> (-50.6002, -52.6435)
  line L674 (-50.6002, -54.3756) -> (-52.1002, -55.2416)
  line L675 (-53.6002, -52.6435) -> (-52.1002, -51.7775)
  line L676 (-52.1002, -55.2416) -> (-53.6002, -54.3756)
  line L677 (-53.6002, -54.3756) -> (-53.6002, -52.6435)
  line L678 (-46.6002, -52.6435) -> (-46.6002, -54.3756)
  line L679 (-48.1002, -51.7775) -> (-46.6002, -52.6435)
  line L680 (-46.6002, -54.3756) -> (-48.1002, -55.2416)
  line L681 (-49.6002, -52.6435) -> (-48.1002, -51.7775)
  line L682 (-48.1002, -55.2416) -> (-49.6002, -54.3756)
  line L683 (-49.6002, -54.3756) -> (-49.6002, -52.6435)
  line L684 (-42.6002, -52.6435) -> (-42.6002, -54.3756)
  line L685 (-44.1002, -51.7775) -> (-42.6002, -52.6435)
  line L686 (-42.6002, -54.3756) -> (-44.1002, -55.2416)
  line L687 (-45.6002, -52.6435) -> (-44.1002, -51.7775)
  line L688 (-44.1002, -55.2416) -> (-45.6002, -54.3756)
  line L689 (-45.6002, -54.3756) -> (-45.6002, -52.6435)
  line L690 (-38.6002, -52.6435) -> (-38.6002, -54.3756)
  line L691 (-40.1002, -51.7775) -> (-38.6002, -52.6435)
  line L692 (-38.6002, -54.3756) -> (-40.1002, -55.2416)
  line L693 (-41.6002, -52.6435) -> (-40.1002, -51.7775)
  line L694 (-40.1002, -55.2416) -> (-41.6002, -54.3756)
  line L695 (-41.6002, -54.3756) -> (-41.6002, -52.6435)
  line L696 (-70.6002, -56.6435) -> (-70.6002, -58.3756)
  line L697 (-72.1002, -55.7775) -> (-70.6002, -56.6435)
  line L698 (-70.6002, -58.3756) -> (-72.1002, -59.2416)
  line L699 (-73.6002, -56.6435) -> (-72.1002, -55.7775)
  line L700 (-72.1002, -59.2416) -> (-73.6002, -58.3756)
  line L701 (-73.6002, -58.3756) -> (-73.6002, -56.6435)
  line L702 (-66.6002, -56.6435) -> (-66.6002, -58.3756)
  line L703 (-68.1002, -55.7775) -> (-66.6002, -56.6435)
  line L704 (-66.6002, -58.3756) -> (-68.1002, -59.2416)
  line L705 (-69.6002, -56.6435) -> (-68.1002, -55.7775)
  line L706 (-68.1002, -59.2416) -> (-69.6002, -58.3756)
  line L707 (-69.6002, -58.3756) -> (-69.6002, -56.6435)
  line L708 (-62.6002, -56.6435) -> (-62.6002, -58.3756)
  line L709 (-64.1002, -55.7775) -> (-62.6002, -56.6435)
  line L710 (-62.6002, -58.3756) -> (-64.1002, -59.2416)
  line L711 (-65.6002, -56.6435) -> (-64.1002, -55.7775)
  line L712 (-64.1002, -59.2416) -> (-65.6002, -58.3756)
  line L713 (-65.6002, -58.3756) -> (-65.6002, -56.6435)
  line L714 (-58.6002, -56.6435) -> (-58.6002, -58.3756)
  line L715 (-60.1002, -55.7775) -> (-58.6002, -56.6435)
  line L716 (-58.6002, -58.3756) -> (-60.1002, -59.2416)
  line L717 (-61.6002, -56.6435) -> (-60.1002, -55.7775)
  line L718 (-60.1002, -59.2416) -> (-61.6002, -58.3756)
  line L719 (-61.6002, -58.3756) -> (-61.6002, -56.6435)
  line L720 (-54.6002, -56.6435) -> (-54.6002, -58.3756)
  line L721 (-56.1002, -55.7775) -> (-54.6002, -56.6435)
  line L722 (-54.6002, -58.3756) -> (-56.1002, -59.2416)
  line L723 (-57.6002, -56.6435) -> (-56.1002, -55.7775)
  line L724 (-56.1002, -59.2416) -> (-57.6002, -58.3756)
  line L725 (-57.6002, -58.3756) -> (-57.6002, -56.6435)
  line L726 (-50.6002, -56.6435) -> (-50.6002, -58.3756)
  line L727 (-52.1002, -55.7775) -> (-50.6002, -56.6435)
  line L728 (-50.6002, -58.3756) -> (-52.1002, -59.2416)
  line L729 (-53.6002, -56.6435) -> (-52.1002, -55.7775)
  line L730 (-52.1002, -59.2416) -> (-53.6002, -58.3756)
  line L731 (-53.6002, -58.3756) -> (-53.6002, -56.6435)
  line L732 (-46.6002, -56.6435) -> (-46.6002, -58.3756)
  line L733 (-48.1002, -55.7775) -> (-46.6002, -56.6435)
  line L734 (-46.6002, -58.3756) -> (-48.1002, -59.2416)
  line L735 (-49.6002, -56.6435) -> (-48.1002, -55.7775)
  line L736 (-48.1002, -59.2416) -> (-49.6002, -58.3756)
  line L737 (-49.6002, -58.3756) -> (-49.6002, -56.6435)
  line L738 (-42.6002, -56.6435) -> (-42.6002, -58.3756)
  line L739 (-44.1002, -55.7775) -> (-42.6002, -56.6435)
  line L740 (-42.6002, -58.3756) -> (-44.1002, -59.2416)
  line L741 (-45.6002, -56.6435) -> (-44.1002, -55.7775)
  line L742 (-44.1002, -59.2416) -> (-45.6002, -58.3756)
  line L743 (-45.6002, -58.3756) -> (-45.6002, -56.6435)
  line L744 (-38.6002, -56.6435) -> (-38.6002, -58.3756)
  line L745 (-40.1002, -55.7775) -> (-38.6002, -56.6435)
  line L746 (-38.6002, -58.3756) -> (-40.1002, -59.2416)
  line L747 (-41.6002, -56.6435) -> (-40.1002, -55.7775)
  line L748 (-40.1002, -59.2416) -> (-41.6002, -58.3756)
  line L749 (-41.6002, -58.3756) -> (-41.6002, -56.6435)
  line L750 (-70.6002, -60.6435) -> (-70.6002, -62.3756)
  line L751 (-72.1002, -59.7775) -> (-70.6002, -60.6435)
  line L752 (-70.6002, -62.3756) -> (-72.1002, -63.2416)
  line L753 (-73.6002, -60.6435) -> (-72.1002, -59.7775)
  line L754 (-72.1002, -63.2416) -> (-73.6002, -62.3756)
  line L755 (-73.6002, -62.3756) -> (-73.6002, -60.6435)
  line L756 (-66.6002, -60.6435) -> (-66.6002, -62.3756)
  line L757 (-68.1002, -59.7775) -> (-66.6002, -60.6435)
  line L758 (-66.6002, -62.3756) -> (-68.1002, -63.2416)
  line L759 (-69.6002, -60.6435) -> (-68.1002, -59.7775)
  line L760 (-68.1002, -63.2416) -> (-69.6002, -62.3756)
  line L761 (-69.6002, -62.3756) -> (-69.6002, -60.6435)
  line L762 (-62.6002, -60.6435) -> (-62.6002, -62.3756)
  line L763 (-64.1002, -59.7775) -> (-62.6002, -60.6435)
  line L764 (-62.6002, -62.3756) -> (-64.1002, -63.2416)
  line L765 (-65.6002, -60.6435) -> (-64.1002, -59.7775)
  line L766 (-64.1002, -63.2416) -> (-65.6002, -62.3756)
  line L767 (-65.6002, -62.3756) -> (-65.6002, -60.6435)
  line L768 (-58.6002, -60.6435) -> (-58.6002, -62.3756)
  line L769 (-60.1002, -59.7775) -> (-58.6002, -60.6435)
  line L770 (-58.6002, -62.3756) -> (-60.1002, -63.2416)
  line L771 (-61.6002, -60.6435) -> (-60.1002, -59.7775)
  line L772 (-60.1002, -63.2416) -> (-61.6002, -62.3756)
  line L773 (-61.6002, -62.3756) -> (-61.6002, -60.6435)
  line L774 (-54.6002, -60.6435) -> (-54.6002, -62.3756)
  line L775 (-56.1002, -59.7775) -> (-54.6002, -60.6435)
  line L776 (-54.6002, -62.3756) -> (-56.1002, -63.2416)
  line L777 (-57.6002, -60.6435) -> (-56.1002, -59.7775)
  line L778 (-56.1002, -63.2416) -> (-57.6002, -62.3756)
  line L779 (-57.6002, -62.3756) -> (-57.6002, -60.6435)
  line L780 (-50.6002, -60.6435) -> (-50.6002, -62.3756)
  line L781 (-52.1002, -59.7775) -> (-50.6002, -60.6435)
  line L782 (-50.6002, -62.3756) -> (-52.1002, -63.2416)
  line L783 (-53.6002, -60.6435) -> (-52.1002, -59.7775)
  line L784 (-52.1002, -63.2416) -> (-53.6002, -62.3756)
  line L785 (-53.6002, -62.3756) -> (-53.6002, -60.6435)
  line L786 (-46.6002, -60.6435) -> (-46.6002, -62.3756)
  line L787 (-48.1002, -59.7775) -> (-46.6002, -60.6435)
  line L788 (-46.6002, -62.3756) -> (-48.1002, -63.2416)
  line L789 (-49.6002, -60.6435) -> (-48.1002, -59.7775)
  line L790 (-48.1002, -63.2416) -> (-49.6002, -62.3756)
  line L791 (-49.6002, -62.3756) -> (-49.6002, -60.6435)
  line L792 (-42.6002, -60.6435) -> (-42.6002, -62.3756)
  line L793 (-44.1002, -59.7775) -> (-42.6002, -60.6435)
  line L794 (-42.6002, -62.3756) -> (-44.1002, -63.2416)
  line L795 (-45.6002, -60.6435) -> (-44.1002, -59.7775)
  line L796 (-44.1002, -63.2416) -> (-45.6002, -62.3756)
  line L797 (-45.6002, -62.3756) -> (-45.6002, -60.6435)
  line L798 (-38.6002, -60.6435) -> (-38.6002, -62.3756)
  line L799 (-40.1002, -59.7775) -> (-38.6002, -60.6435)
  line L800 (-38.6002, -62.3756) -> (-40.1002, -63.2416)
  line L801 (-41.6002, -60.6435) -> (-40.1002, -59.7775)
  line L802 (-40.1002, -63.2416) -> (-41.6002, -62.3756)
  line L803 (-41.6002, -62.3756) -> (-41.6002, -60.6435)
  line L804 (-70.6002, -64.6435) -> (-70.6002, -66.3756)
  line L805 (-72.1002, -63.7775) -> (-70.6002, -64.6435)
  line L806 (-70.6002, -66.3756) -> (-72.1002, -67.2416)
  line L807 (-73.6002, -64.6435) -> (-72.1002, -63.7775)
  line L808 (-72.1002, -67.2416) -> (-73.6002, -66.3756)
  line L809 (-73.6002, -66.3756) -> (-73.6002, -64.6435)
  line L810 (-66.6002, -64.6435) -> (-66.6002, -66.3756)
  line L811 (-68.1002, -63.7775) -> (-66.6002, -64.6435)
  line L812 (-66.6002, -66.3756) -> (-68.1002, -67.2416)
  line L813 (-69.6002, -64.6435) -> (-68.1002, -63.7775)
  line L814 (-68.1002, -67.2416) -> (-69.6002, -66.3756)
  line L815 (-69.6002, -66.3756) -> (-69.6002, -64.6435)
  line L816 (-62.6002, -64.6435) -> (-62.6002, -66.3756)
  line L817 (-64.1002, -63.7775) -> (-62.6002, -64.6435)
  line L818 (-62.6002, -66.3756) -> (-64.1002, -67.2416)
  line L819 (-65.6002, -64.6435) -> (-64.1002, -63.7775)
  line L820 (-64.1002, -67.2416) -> (-65.6002, -66.3756)
  line L821 (-65.6002, -66.3756) -> (-65.6002, -64.6435)
  line L822 (-58.6002, -64.6435) -> (-58.6002, -66.3756)
  line L823 (-60.1002, -63.7775) -> (-58.6002, -64.6435)
  line L824 (-58.6002, -66.3756) -> (-60.1002, -67.2416)
  line L825 (-61.6002, -64.6435) -> (-60.1002, -63.7775)
  line L826 (-60.1002, -67.2416) -> (-61.6002, -66.3756)
  line L827 (-61.6002, -66.3756) -> (-61.6002, -64.6435)
  line L828 (-54.6002, -64.6435) -> (-54.6002, -66.3756)
  line L829 (-56.1002, -63.7775) -> (-54.6002, -64.6435)
  line L830 (-54.6002, -66.3756) -> (-56.1002, -67.2416)
  line L831 (-57.6002, -64.6435) -> (-56.1002, -63.7775)
  line L832 (-56.1002, -67.2416) -> (-57.6002, -66.3756)
  line L833 (-57.6002, -66.3756) -> (-57.6002, -64.6435)
  line L834 (-50.6002, -64.6435) -> (-50.6002, -66.3756)
  line L835 (-52.1002, -63.7775) -> (-50.6002, -64.6435)
  line L836 (-50.6002, -66.3756) -> (-52.1002, -67.2416)
  line L837 (-53.6002, -64.6435) -> (-52.1002, -63.7775)
  line L838 (-52.1002, -67.2416) -> (-53.6002, -66.3756)
  line L839 (-53.6002, -66.3756) -> (-53.6002, -64.6435)
  line L840 (-46.6002, -64.6435) -> (-46.6002, -66.3756)
  line L841 (-48.1002, -63.7775) -> (-46.6002, -64.6435)
  line L842 (-46.6002, -66.3756) -> (-48.1002, -67.2416)
  line L843 (-49.6002, -64.6435) -> (-48.1002, -63.7775)